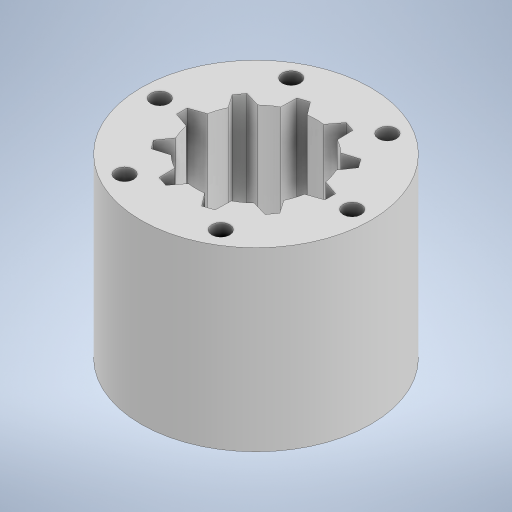
# Autodesk Inventor part: Wrist Arm Plates
Saved by Autodesk Inventor 2024 (Build 280153000, 153)
## iProperties
Created: 2023-06-27
Part Number: Wrist Arm Plates
Material: Generic
Document SubType Name: Modeling
Designer: t205b
Density: 1 g/cm^3
Appearance: Default
Author: t205b
Autodesk Inventor part; units mm, degrees
ref_plane "YZ Plane" through (0, 0, 0) normal (1, 0, 0) x (0, 1, 0)
ref_plane "XZ Plane" through (0, 0, 0) normal (0, 1, 0) x (-1, 0, 0)
ref_plane "XY Plane" through (0, 0, 0) normal (0, 0, 1) x (1, 0, 0)
sketch "Sketch1" plane through (0, 0, 0) normal (0, 1, 0) x (-1, 0, 0)
  circle A0 centre (0, 0) radius 17
  line L0 (16.7332, -3) -> (21, -1.5)
  line L1 (21, -1.5) -> (21, 1.5)
  line L2 (21, 1.5) -> (16.7332, 3)
  line L3 (15.3008, 7.4085) -> (17.871, 11.13)
  line L4 (17.871, 11.13) -> (16.1077, 13.557)
  line L5 (16.1077, 13.557) -> (11.7741, 12.2626)
  line L6 (8.024, 14.9872) -> (7.9159, 19.5087)
  line L7 (7.9159, 19.5087) -> (5.0628, 20.4357)
  line L8 (5.0628, 20.4357) -> (2.3177, 16.8413)
  line L9 (-2.3177, 16.8413) -> (-5.0628, 20.4357)
  line L10 (-5.0628, 20.4357) -> (-7.9159, 19.5087)
  line L11 (-7.9159, 19.5087) -> (-8.024, 14.9872)
  line L12 (-11.7741, 12.2626) -> (-16.1077, 13.557)
  line L13 (-16.1077, 13.557) -> (-17.871, 11.13)
  line L14 (-17.871, 11.13) -> (-15.3008, 7.4085)
  line L15 (-16.7332, 3) -> (-21, 1.5)
  line L16 (-21, 1.5) -> (-21, -1.5)
  line L17 (-21, -1.5) -> (-16.7332, -3)
  line L18 (-15.3008, -7.4085) -> (-17.871, -11.13)
  line L19 (-17.871, -11.13) -> (-16.1077, -13.557)
  line L20 (-16.1077, -13.557) -> (-11.7741, -12.2626)
  line L21 (-8.024, -14.9872) -> (-7.9159, -19.5087)
  line L22 (-7.9159, -19.5087) -> (-5.0628, -20.4357)
  line L23 (-5.0628, -20.4357) -> (-2.3177, -16.8413)
  line L24 (2.3177, -16.8413) -> (5.0628, -20.4357)
  line L25 (5.0628, -20.4357) -> (7.9159, -19.5087)
  line L26 (7.9159, -19.5087) -> (8.024, -14.9872)
  line L27 (11.7741, -12.2626) -> (16.1077, -13.557)
  line L28 (16.1077, -13.557) -> (17.871, -11.13)
  line L29 (17.871, -11.13) -> (15.3008, -7.4085)
  dimension "d0" = 34
  dimension "d1" = 3
  dimension "d2" = 6
  dimension "d3" = 4
  dimension "d4" = 109.369
  dimension "d5" = 109.369
  dimension "d8" = 360
  constraints: 60 end point, 2 point on circle, 1 centre point, 1 coincident, 1 equal length, 1 vertical, 71 other
  measures "d0" diameter of A0
  measures "d1" distance of L0.end L1.end
  measures "d2" distance of L2.end L0.start
  measures "d3" distance edge to line of A0 L1
  measures "d4" angle of L2 L1
  measures "d5" angle of L0 L1
extrude "Extrusion1" add sketch "Sketch1" along normal blind 5
sketch "Sketch2" plane through (0, 5, 0) normal (0, 1, 0) x (1, 0, 0)
  line L0 (-15.3008, -7.4085) -> (-17.871, -11.13) projected
  line L1 (-17.871, -11.13) -> (-16.1077, -13.557) projected
  line L2 (-16.1077, -13.557) -> (-11.7741, -12.2626) projected
  arc A0 (-11.7741, -12.2626) -> (-8.024, -14.9872) centre (0, 0) ccw projected
  line L3 (-8.024, -14.9872) -> (-7.9159, -19.5087) projected
  line L4 (-7.9159, -19.5087) -> (-5.0628, -20.4357) projected
  line L5 (-5.0628, -20.4357) -> (-2.3177, -16.8413) projected
  arc A1 (-2.3177, -16.8413) -> (2.3177, -16.8413) centre (0, 0) ccw projected
  line L6 (2.3177, -16.8413) -> (5.0628, -20.4357) projected
  line L7 (5.0628, -20.4357) -> (7.9159, -19.5087) projected
  line L8 (7.9159, -19.5087) -> (8.024, -14.9872) projected
  arc A2 (8.024, -14.9872) -> (11.7741, -12.2626) centre (0, 0) ccw projected
  line L9 (11.7741, -12.2626) -> (16.1077, -13.557) projected
  line L10 (16.1077, -13.557) -> (17.871, -11.13) projected
  line L11 (17.871, -11.13) -> (15.3008, -7.4085) projected
  arc A3 (15.3008, -7.4085) -> (16.7332, -3) centre (0, 0) ccw projected
  line L12 (16.7332, -3) -> (21, -1.5) projected
  line L13 (21, -1.5) -> (21, 1.5) projected
  line L14 (21, 1.5) -> (16.7332, 3) projected
  arc A4 (16.7332, 3) -> (15.3008, 7.4085) centre (0, 0) ccw projected
  line L15 (15.3008, 7.4085) -> (17.871, 11.13) projected
  line L16 (17.871, 11.13) -> (16.1077, 13.557) projected
  line L17 (16.1077, 13.557) -> (11.7741, 12.2626) projected
  arc A5 (11.7741, 12.2626) -> (8.024, 14.9872) centre (0, 0) ccw projected
  line L18 (8.024, 14.9872) -> (7.9159, 19.5087) projected
  line L19 (7.9159, 19.5087) -> (5.0628, 20.4357) projected
  line L20 (5.0628, 20.4357) -> (2.3177, 16.8413) projected
  arc A6 (2.3177, 16.8413) -> (-2.3177, 16.8413) centre (0, 0) ccw projected
  line L21 (-2.3177, 16.8413) -> (-5.0628, 20.4357) projected
  line L22 (-5.0628, 20.4357) -> (-7.9159, 19.5087) projected
  line L23 (-7.9159, 19.5087) -> (-8.024, 14.9872) projected
  arc A7 (-8.024, 14.9872) -> (-11.7741, 12.2626) centre (0, 0) ccw projected
  line L24 (-11.7741, 12.2626) -> (-16.1077, 13.557) projected
  line L25 (-16.1077, 13.557) -> (-17.871, 11.13) projected
  line L26 (-17.871, 11.13) -> (-15.3008, 7.4085) projected
  arc A8 (-15.3008, 7.4085) -> (-16.7332, 3) centre (0, 0) ccw projected
  line L27 (-16.7332, 3) -> (-21, 1.5) projected
  line L28 (-21, 1.5) -> (-21, -1.5) projected
  line L29 (-21, -1.5) -> (-16.7332, -3) projected
  arc A9 (-16.7332, -3) -> (-15.3008, -7.4085) centre (0, 0) ccw projected
extrude "Extrusion2" add sketch "Sketch2" along normal blind 500
sketch "Sketch3" plane through (0, 505, 0) normal (0, 1, 0) x (1, 0, 0)
  circle A0 centre (0, 0) radius 4
  dimension "d14" = 8
  constraints: 1 centre point, 1 coincident
  measures "d14" diameter of A0
extrude "Extrusion3" cut sketch "Sketch3" against normal blind 528.7
sketch "Sketch4" plane through (0, 505, 0) normal (0, 1, 0) x (1, 0, 0)
  circle A0 centre (0, 0) radius 4 projected
  line L0 (-17.871, -11.13) -> (-16.1077, -13.557) projected
  line L1 (-16.1077, -13.557) -> (-11.7741, -12.2626) projected
  arc A1 (-11.7741, -12.2626) -> (-8.024, -14.9872) centre (0, 0) ccw projected
  line L2 (-8.024, -14.9872) -> (-7.9159, -19.5087) projected
  line L3 (-7.9159, -19.5087) -> (-5.0628, -20.4357) projected
  line L4 (-5.0628, -20.4357) -> (-2.3177, -16.8413) projected
  arc A2 (-2.3177, -16.8413) -> (2.3177, -16.8413) centre (0, 0) ccw projected
  line L5 (2.3177, -16.8413) -> (5.0628, -20.4357) projected
  line L6 (5.0628, -20.4357) -> (7.9159, -19.5087) projected
  line L7 (7.9159, -19.5087) -> (8.024, -14.9872) projected
  arc A3 (8.024, -14.9872) -> (11.7741, -12.2626) centre (0, 0) ccw projected
  line L8 (11.7741, -12.2626) -> (16.1077, -13.557) projected
  line L9 (16.1077, -13.557) -> (17.871, -11.13) projected
  line L10 (17.871, -11.13) -> (15.3008, -7.4085) projected
  arc A4 (15.3008, -7.4085) -> (16.7332, -3) centre (0, 0) ccw projected
  line L11 (16.7332, -3) -> (21, -1.5) projected
  line L12 (21, -1.5) -> (21, 1.5) projected
  line L13 (21, 1.5) -> (16.7332, 3) projected
  arc A5 (16.7332, 3) -> (15.3008, 7.4085) centre (0, 0) ccw projected
  line L14 (15.3008, 7.4085) -> (17.871, 11.13) projected
  line L15 (17.871, 11.13) -> (16.1077, 13.557) projected
  line L16 (16.1077, 13.557) -> (11.7741, 12.2626) projected
  arc A6 (11.7741, 12.2626) -> (8.024, 14.9872) centre (0, 0) ccw projected
  line L17 (8.024, 14.9872) -> (7.9159, 19.5087) projected
  line L18 (7.9159, 19.5087) -> (5.0628, 20.4357) projected
  line L19 (5.0628, 20.4357) -> (2.3177, 16.8413) projected
  arc A7 (2.3177, 16.8413) -> (-2.3177, 16.8413) centre (0, 0) ccw projected
  line L20 (-2.3177, 16.8413) -> (-5.0628, 20.4357) projected
  line L21 (-5.0628, 20.4357) -> (-7.9159, 19.5087) projected
  line L22 (-7.9159, 19.5087) -> (-8.024, 14.9872) projected
  arc A8 (-8.024, 14.9872) -> (-11.7741, 12.2626) centre (0, 0) ccw projected
  line L23 (-11.7741, 12.2626) -> (-16.1077, 13.557) projected
  line L24 (-16.1077, 13.557) -> (-17.871, 11.13) projected
  line L25 (-17.871, 11.13) -> (-15.3008, 7.4085) projected
  arc A9 (-15.3008, 7.4085) -> (-16.7332, 3) centre (0, 0) ccw projected
  line L26 (-16.7332, 3) -> (-21, 1.5) projected
  line L27 (-21, 1.5) -> (-21, -1.5) projected
  line L28 (-21, -1.5) -> (-16.7332, -3) projected
  arc A10 (-16.7332, -3) -> (-15.3008, -7.4085) centre (0, 0) ccw projected
  line L29 (-15.3008, -7.4085) -> (-17.871, -11.13) projected
extrude "Extrusion4" cut sketch "Sketch4" against normal blind 449.2 contours A0 | L29 A10 L28 L27 L26 A9 L25 L24 L23 A8 L22 L21 L20 A7 L19 L18 L17 A6 L16 L15 L14 A5 L13 L12 L11 A4 L10 L9 L8 A3 L7 L6 L5 A2 L4 L3 L2 A1 L1 L0
sketch "Sketch5" plane through (0, 55.8, 0) normal (0, 1, 0) x (1, 0, 0)
  circle A0 centre (0, 0) radius 4 projected
  line L0 (-11.7741, -12.2626) -> (-16.1077, -13.557) projected
  arc A1 (-11.7741, -12.2626) -> (-8.024, -14.9872) centre (0, 0) ccw projected
  line L1 (-7.9159, -19.5087) -> (-8.024, -14.9872) projected
  line L2 (-5.0628, -20.4357) -> (-7.9159, -19.5087) projected
  line L3 (-2.3177, -16.8413) -> (-5.0628, -20.4357) projected
  arc A2 (-2.3177, -16.8413) -> (2.3177, -16.8413) centre (0, 0) ccw projected
  line L4 (5.0628, -20.4357) -> (2.3177, -16.8413) projected
  line L5 (7.9159, -19.5087) -> (5.0628, -20.4357) projected
  line L6 (8.024, -14.9872) -> (7.9159, -19.5087) projected
  arc A3 (8.024, -14.9872) -> (11.7741, -12.2626) centre (0, 0) ccw projected
  line L7 (16.1077, -13.557) -> (11.7741, -12.2626) projected
  line L8 (17.871, -11.13) -> (16.1077, -13.557) projected
  line L9 (15.3008, -7.4085) -> (17.871, -11.13) projected
  arc A4 (15.3008, -7.4085) -> (16.7332, -3) centre (0, 0) ccw projected
  line L10 (21, -1.5) -> (16.7332, -3) projected
  line L11 (21, 1.5) -> (21, -1.5) projected
  line L12 (16.7332, 3) -> (21, 1.5) projected
  arc A5 (16.7332, 3) -> (15.3008, 7.4085) centre (0, 0) ccw projected
  line L13 (17.871, 11.13) -> (15.3008, 7.4085) projected
  line L14 (16.1077, 13.557) -> (17.871, 11.13) projected
  line L15 (11.7741, 12.2626) -> (16.1077, 13.557) projected
  arc A6 (11.7741, 12.2626) -> (8.024, 14.9872) centre (0, 0) ccw projected
  line L16 (7.9159, 19.5087) -> (8.024, 14.9872) projected
  line L17 (5.0628, 20.4357) -> (7.9159, 19.5087) projected
  line L18 (2.3177, 16.8413) -> (5.0628, 20.4357) projected
  arc A7 (2.3177, 16.8413) -> (-2.3177, 16.8413) centre (0, 0) ccw projected
  line L19 (-5.0628, 20.4357) -> (-2.3177, 16.8413) projected
  line L20 (-7.9159, 19.5087) -> (-5.0628, 20.4357) projected
  line L21 (-8.024, 14.9872) -> (-7.9159, 19.5087) projected
  arc A8 (-8.024, 14.9872) -> (-11.7741, 12.2626) centre (0, 0) ccw projected
  line L22 (-16.1077, 13.557) -> (-11.7741, 12.2626) projected
  line L23 (-17.871, 11.13) -> (-16.1077, 13.557) projected
  line L24 (-15.3008, 7.4085) -> (-17.871, 11.13) projected
  arc A9 (-15.3008, 7.4085) -> (-16.7332, 3) centre (0, 0) ccw projected
  line L25 (-21, 1.5) -> (-16.7332, 3) projected
  line L26 (-21, -1.5) -> (-21, 1.5) projected
  line L27 (-16.7332, -3) -> (-21, -1.5) projected
  arc A10 (-16.7332, -3) -> (-15.3008, -7.4085) centre (0, 0) ccw projected
  line L28 (-17.871, -11.13) -> (-15.3008, -7.4085) projected
  line L29 (-16.1077, -13.557) -> (-17.871, -11.13) projected
extrude "Extrusion5" cut sketch "Sketch5" against normal blind 5.8
sketch "Sketch6" plane through (0, 50, 0) normal (0, 1, 0) x (1, 0, 0)
  circle A0 centre (0, 0) radius 45
  line L0 (5.0628, -20.4357) -> (2.3177, -16.8413) projected
  line L1 (7.9159, -19.5087) -> (5.0628, -20.4357) projected
  line L2 (8.024, -14.9872) -> (7.9159, -19.5087) projected
  arc A1 (8.024, -14.9872) -> (11.7741, -12.2626) centre (0, 0) ccw projected
  line L3 (16.1077, -13.557) -> (11.7741, -12.2626) projected
  line L4 (17.871, -11.13) -> (16.1077, -13.557) projected
  line L5 (15.3008, -7.4085) -> (17.871, -11.13) projected
  arc A2 (15.3008, -7.4085) -> (16.7332, -3) centre (0, 0) ccw projected
  line L6 (21, -1.5) -> (16.7332, -3) projected
  line L7 (21, 1.5) -> (21, -1.5) projected
  line L8 (16.7332, 3) -> (21, 1.5) projected
  arc A3 (16.7332, 3) -> (15.3008, 7.4085) centre (0, 0) ccw projected
  line L9 (17.871, 11.13) -> (15.3008, 7.4085) projected
  line L10 (16.1077, 13.557) -> (17.871, 11.13) projected
  line L11 (11.7741, 12.2626) -> (16.1077, 13.557) projected
  arc A4 (11.7741, 12.2626) -> (8.024, 14.9872) centre (0, 0) ccw projected
  line L12 (7.9159, 19.5087) -> (8.024, 14.9872) projected
  line L13 (5.0628, 20.4357) -> (7.9159, 19.5087) projected
  line L14 (2.3177, 16.8413) -> (5.0628, 20.4357) projected
  arc A5 (2.3177, 16.8413) -> (-2.3177, 16.8413) centre (0, 0) ccw projected
  line L15 (-5.0628, 20.4357) -> (-2.3177, 16.8413) projected
  line L16 (-7.9159, 19.5087) -> (-5.0628, 20.4357) projected
  line L17 (-8.024, 14.9872) -> (-7.9159, 19.5087) projected
  arc A6 (-8.024, 14.9872) -> (-11.7741, 12.2626) centre (0, 0) ccw projected
  line L18 (-16.1077, 13.557) -> (-11.7741, 12.2626) projected
  line L19 (-17.871, 11.13) -> (-16.1077, 13.557) projected
  line L20 (-15.3008, 7.4085) -> (-17.871, 11.13) projected
  arc A7 (-15.3008, 7.4085) -> (-16.7332, 3) centre (0, 0) ccw projected
  line L21 (-21, 1.5) -> (-16.7332, 3) projected
  line L22 (-21, -1.5) -> (-21, 1.5) projected
  line L23 (-16.7332, -3) -> (-21, -1.5) projected
  arc A8 (-16.7332, -3) -> (-15.3008, -7.4085) centre (0, 0) ccw projected
  line L24 (-17.871, -11.13) -> (-15.3008, -7.4085) projected
  line L25 (-16.1077, -13.557) -> (-17.871, -11.13) projected
  line L26 (-11.7741, -12.2626) -> (-16.1077, -13.557) projected
  arc A9 (-11.7741, -12.2626) -> (-8.024, -14.9872) centre (0, 0) ccw projected
  line L27 (-7.9159, -19.5087) -> (-8.024, -14.9872) projected
  line L28 (-5.0628, -20.4357) -> (-7.9159, -19.5087) projected
  line L29 (-2.3177, -16.8413) -> (-5.0628, -20.4357) projected
  arc A10 (-2.3177, -16.8413) -> (2.3177, -16.8413) centre (0, 0) ccw projected
  circle A11 centre (0, 0) radius 4 projected
  dimension "d21" = 90
  constraints: 1 centre point, 1 coincident
  measures "d21" diameter of A0
extrude "Extrusion6" add sketch "Sketch6" along normal blind 50 contours A0
sketch "Sketch7" plane through (0, 100, 0) normal (0, 1, 0) x (1, 0, 0)
  circle A0 centre (0, 0) radius 45 projected
  line L0 (8.024, -14.9872) -> (7.9159, -19.5087) projected
  line L1 (7.9159, -19.5087) -> (5.0628, -20.4357) projected
  line L2 (5.0628, -20.4357) -> (2.3177, -16.8413) projected
  arc A1 (-2.3177, -16.8413) -> (2.3177, -16.8413) centre (0, 0) ccw projected
  line L3 (-2.3177, -16.8413) -> (-5.0628, -20.4357) projected
  line L4 (-5.0628, -20.4357) -> (-7.9159, -19.5087) projected
  line L5 (-7.9159, -19.5087) -> (-8.024, -14.9872) projected
  arc A2 (-11.7741, -12.2626) -> (-8.024, -14.9872) centre (0, 0) ccw projected
  line L6 (-11.7741, -12.2626) -> (-16.1077, -13.557) projected
  line L7 (-16.1077, -13.557) -> (-17.871, -11.13) projected
  line L8 (-17.871, -11.13) -> (-15.3008, -7.4085) projected
  arc A3 (-16.7332, -3) -> (-15.3008, -7.4085) centre (0, 0) ccw projected
  line L9 (-16.7332, -3) -> (-21, -1.5) projected
  line L10 (-21, -1.5) -> (-21, 1.5) projected
  line L11 (-21, 1.5) -> (-16.7332, 3) projected
  arc A4 (-15.3008, 7.4085) -> (-16.7332, 3) centre (0, 0) ccw projected
  line L12 (-15.3008, 7.4085) -> (-17.871, 11.13) projected
  line L13 (-17.871, 11.13) -> (-16.1077, 13.557) projected
  line L14 (-16.1077, 13.557) -> (-11.7741, 12.2626) projected
  arc A5 (-8.024, 14.9872) -> (-11.7741, 12.2626) centre (0, 0) ccw projected
  line L15 (-8.024, 14.9872) -> (-7.9159, 19.5087) projected
  line L16 (-7.9159, 19.5087) -> (-5.0628, 20.4357) projected
  line L17 (-5.0628, 20.4357) -> (-2.3177, 16.8413) projected
  arc A6 (2.3177, 16.8413) -> (-2.3177, 16.8413) centre (0, 0) ccw projected
  line L18 (2.3177, 16.8413) -> (5.0628, 20.4357) projected
  line L19 (5.0628, 20.4357) -> (7.9159, 19.5087) projected
  line L20 (7.9159, 19.5087) -> (8.024, 14.9872) projected
  arc A7 (11.7741, 12.2626) -> (8.024, 14.9872) centre (0, 0) ccw projected
  line L21 (11.7741, 12.2626) -> (16.1077, 13.557) projected
  line L22 (16.1077, 13.557) -> (17.871, 11.13) projected
  line L23 (17.871, 11.13) -> (15.3008, 7.4085) projected
  arc A8 (16.7332, 3) -> (15.3008, 7.4085) centre (0, 0) ccw projected
  line L24 (16.7332, 3) -> (21, 1.5) projected
  line L25 (21, 1.5) -> (21, -1.5) projected
  line L26 (21, -1.5) -> (16.7332, -3) projected
  arc A9 (15.3008, -7.4085) -> (16.7332, -3) centre (0, 0) ccw projected
  line L27 (15.3008, -7.4085) -> (17.871, -11.13) projected
  line L28 (17.871, -11.13) -> (16.1077, -13.557) projected
  line L29 (16.1077, -13.557) -> (11.7741, -12.2626) projected
  arc A10 (8.024, -14.9872) -> (11.7741, -12.2626) centre (0, 0) ccw projected
  circle A11 centre (0, 0) radius 32.5
  dimension "d24" = 65
  constraints: 1 centre point, 1 coincident
  measures "d24" diameter of A11
extrude "Extrusion7" cut sketch "Sketch7" against normal blind 75.4125 contours A0
sketch "Sketch8" plane through (0, 0, 0) normal (0, -1, 0) x (1, 0, 0)
  circle A0 centre (0, 0) radius 4 projected
  line L0 (-15.3008, 7.4085) -> (-17.871, 11.13) projected
  arc A1 (-15.3008, 7.4085) -> (-16.7332, 3) centre (0, 0) ccw projected
  line L1 (-21, 1.5) -> (-16.7332, 3) projected
  line L2 (-21, -1.5) -> (-21, 1.5) projected
  line L3 (-16.7332, -3) -> (-21, -1.5) projected
  arc A2 (-16.7332, -3) -> (-15.3008, -7.4085) centre (0, 0) ccw projected
  line L4 (-17.871, -11.13) -> (-15.3008, -7.4085) projected
  line L5 (-16.1077, -13.557) -> (-17.871, -11.13) projected
  line L6 (-11.7741, -12.2626) -> (-16.1077, -13.557) projected
  arc A3 (-11.7741, -12.2626) -> (-8.024, -14.9872) centre (0, 0) ccw projected
  line L7 (-7.9159, -19.5087) -> (-8.024, -14.9872) projected
  line L8 (-5.0628, -20.4357) -> (-7.9159, -19.5087) projected
  line L9 (-2.3177, -16.8413) -> (-5.0628, -20.4357) projected
  arc A4 (-2.3177, -16.8413) -> (2.3177, -16.8413) centre (0, 0) ccw projected
  line L10 (5.0628, -20.4357) -> (2.3177, -16.8413) projected
  line L11 (7.9159, -19.5087) -> (5.0628, -20.4357) projected
  line L12 (8.024, -14.9872) -> (7.9159, -19.5087) projected
  arc A5 (8.024, -14.9872) -> (11.7741, -12.2626) centre (0, 0) ccw projected
  line L13 (16.1077, -13.557) -> (11.7741, -12.2626) projected
  line L14 (17.871, -11.13) -> (16.1077, -13.557) projected
  line L15 (15.3008, -7.4085) -> (17.871, -11.13) projected
  arc A6 (15.3008, -7.4085) -> (16.7332, -3) centre (0, 0) ccw projected
  line L16 (21, -1.5) -> (16.7332, -3) projected
  line L17 (21, 1.5) -> (21, -1.5) projected
  line L18 (16.7332, 3) -> (21, 1.5) projected
  arc A7 (16.7332, 3) -> (15.3008, 7.4085) centre (0, 0) ccw projected
  line L19 (17.871, 11.13) -> (15.3008, 7.4085) projected
  line L20 (16.1077, 13.557) -> (17.871, 11.13) projected
  line L21 (11.7741, 12.2626) -> (16.1077, 13.557) projected
  arc A8 (11.7741, 12.2626) -> (8.024, 14.9872) centre (0, 0) ccw projected
  line L22 (7.9159, 19.5087) -> (8.024, 14.9872) projected
  line L23 (5.0628, 20.4357) -> (7.9159, 19.5087) projected
  line L24 (2.3177, 16.8413) -> (5.0628, 20.4357) projected
  arc A9 (2.3177, 16.8413) -> (-2.3177, 16.8413) centre (0, 0) ccw projected
  line L25 (-5.0628, 20.4357) -> (-2.3177, 16.8413) projected
  line L26 (-7.9159, 19.5087) -> (-5.0628, 20.4357) projected
  line L27 (-8.024, 14.9872) -> (-7.9159, 19.5087) projected
  arc A10 (-8.024, 14.9872) -> (-11.7741, 12.2626) centre (0, 0) ccw projected
  line L28 (-16.1077, 13.557) -> (-11.7741, 12.2626) projected
  line L29 (-17.871, 11.13) -> (-16.1077, 13.557) projected
extrude "Extrusion8" cut sketch "Sketch8" against normal up to surface (50 mm away)
sketch "Sketch9" plane through (0, 100, 0) normal (0, 1, 0) x (1, 0, 0)
  circle A0 centre (-27.2136, 0) radius 2.5527
  circle A1 centre (0, 0) radius 27.2136
  circle A2 centre (-13.6068, -23.5677) radius 2.5527
  circle A3 centre (0, 0) radius 27.2136
  circle A4 centre (13.6068, -23.5677) radius 2.5527
  circle A5 centre (0, 0) radius 27.2136
  circle A6 centre (27.2136, 0) radius 2.5527
  circle A7 centre (0, 0) radius 27.2136
  circle A8 centre (13.6068, 23.5677) radius 2.5527
  circle A9 centre (0, 0) radius 27.2136
  circle A10 centre (-13.6068, 23.5677) radius 2.5527
  circle A11 centre (0, 0) radius 27.2136
  dimension "d29" = 5.1054
  dimension "d32" = 360
  constraints: 6 centre point, 3 coincident, 2 horizontal alignment, 39 other
  measures "d29" diameter of A0
extrude "Extrusion9" cut sketch "Sketch9" against normal blind 74.1375 contours A0 A1 | A1 A0 | A10 A1 | A1 A10 | A2 A1 | A1 A2 | A8 A1 | A1 A8 | A4 A1 | A1 A4 | A6 A1 | A1 A6
equation "\"d4\" = d5"
body "Solid1"
